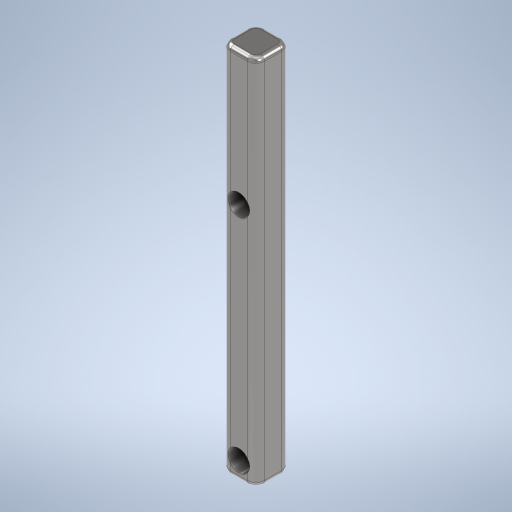
# Autodesk Inventor part: wedgec
Saved by Autodesk Inventor 2023 (Build 270158000, 158)
## iProperties
Created: 2022-05-23
Part Number: wedgec
Material: Stainless Steel
Document SubType Name: Modeling
Designer: aaron
Density: 8 g/cm^3
Appearance: Semi-Polished
Author: aaron
Autodesk Inventor part; units mm, degrees
ref_plane "YZ Plane" through (0, 0, 0) normal (1, 0, 0) x (0, 1, 0)
ref_plane "XZ Plane" through (0, 0, 0) normal (0, 1, 0) x (-1, 0, 0)
ref_plane "XY Plane" through (0, 0, 0) normal (0, 0, 1) x (1, 0, 0)
sketch "Sketch1" plane through (0, 0, 0) normal (0, 1, 0) x (-1, 0, 0)
  line L0 (-3.175, -3.175) -> (3.175, -3.175)
  line L1 (3.175, -3.175) -> (3.175, 3.175)
  line L2 (3.175, 3.175) -> (-3.175, 3.175)
  line L3 (-3.175, 3.175) -> (-3.175, -3.175)
  line L4 (-3.175, -3.175) -> (3.175, 3.175) construction
  line L5 (3.175, -3.175) -> (-3.175, 3.175) construction
  point P0 (0, 0)
  dimension "d0" = 6.35
  dimension "d1" = 6.35
  constraints: 12 end point, 2 midpoint, 2 parallel, 1 horizontal, 1 perpendicular
  measures "d0" distance of L2.end L1.end
  measures "d1" distance of L1.end L0.end
extrude "Extrusion1" add sketch "Sketch1" along normal blind 68.58
fillet "Fillet1" radius 1.5875 4 edges at (3.175, 34.29, 3.175) (3.175, 34.29, -3.175) (-3.175, 34.29, -3.175) (-3.175, 34.29, 3.175)
fillet "Fillet2" radius 0.7937 16 edges at (2.71, 0, -2.71) (0, 0, -3.175) (-2.71, 0, -2.71) (-3.175, 0, 0) (-2.71, 0, 2.71) (0, 0, 3.175) (2.71, 0, 2.71) (3.175, 0, 0) (2.71, 68.58, -2.71) (0, 68.58, -3.175) (-2.71, 68.58, -2.71) (-3.175, 68.58, 0) (-2.71, 68.58, 2.71) (0, 68.58, 3.175) (2.71, 68.58, 2.71) (3.175, 68.58, 0)
sketch "Sketch2" plane through (-1.5875, 67.7863, 3.175) normal (0, 0, 1) x (1, 0, 0)
  circle A0 centre (1.5875, -64.6113) radius 1.9844
  line L0 (0, -67.7863) -> (3.175, -67.7863) projected
  point P0 (1.5875, -67.7863)
  dimension "d6" = 3.9688
  dimension "d7" = 3.175
  constraints: 1 centre point
  measures "d6" diameter of A0
  measures "d7" distance from line of L0 A0.centre
extrude "Extrusion2" cut sketch "Sketch2" against normal blind 50.8
sketch "Sketch3" plane through (-1.5875, 67.7863, 3.175) normal (0, 0, 1) x (1, 0, 0)
  circle A0 centre (1.5875, -23.7173) radius 1.9844
  arc A1 (3.175, -63.4206) -> (0, -63.4206) centre (1.5875, -64.6113) ccw projected
  point P0 (1.5875, -67.7863)
  dimension "d10" = 3.9688
  dimension "d11" = 40.894
  constraints: 1 centre point
  measures "d10" diameter of A0
  measures "d11" distance of A1.centre A0.centre
extrude "Extrusion3" cut sketch "Sketch3" against normal blind 50.8
body "Solid1"
